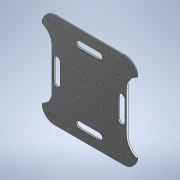
# Autodesk Inventor part: payload_bay_square_FC
Saved by Autodesk Inventor 2022 (Build 260153000, 153)
## iProperties
Created: 2020-02-18
Part Number: payload_bay_square_FC
Material: ABS Plastic
Document SubType Name: Modeling
Designer: Krishna Makhija
Density: 1.06 g/cm^3
Appearance: Smooth - White
Author: Krishna Makhija
Autodesk Inventor part; units mm, degrees
ref_plane "YZ Plane" through (0, 0, 0) normal (1, 0, 0) x (0, 1, 0)
ref_plane "XZ Plane" through (0, 0, 0) normal (0, 1, 0) x (-1, 0, 0)
ref_plane "XY Plane" through (0, 0, 0) normal (0, 0, 1) x (1, 0, 0)
sketch "Sketch1" plane through (0, 0, 0) normal (0, 0, 1) x (1, 0, 0)
  point P0 (0, 0)
sketch "Sketch2" plane through (0, 0, 0) normal (0, 0, 1) x (1, 0, 0)
  line L0 (94.9998, -95.0001) -> (-94.9998, -95.0001)
  line L1 (-94.9998, -95.0001) -> (-94.9998, 95.0001)
  line L2 (-94.9998, 95.0001) -> (94.9998, 95.0001)
  line L3 (94.9998, 95.0001) -> (94.9998, -95.0001)
  line L4 (94.9998, -95.0001) -> (-94.9998, 95.0001) construction
  line L5 (-94.9998, -95.0001) -> (94.9998, 95.0001) construction
  point P0 (0, 0)
  constraints: 12 end point, 2 midpoint, 2 parallel, 1 horizontal, 1 perpendicular
extrude "Extrusion1" add sketch "Sketch2" along normal blind 3
sketch "Sketch3" plane through (0, 0, 3) normal (0, 0, 1) x (1, 0, 0)
  circle A0 centre (70, 80) radius 1.5001
  circle A1 centre (70, -80) radius 1.5001
  circle A2 centre (-70, 80) radius 1.5001
  circle A3 centre (-70, -80) radius 1.5001
  constraints: 4 centre point
extrude "Extrusion2" cut sketch "Sketch3" against normal blind 3
fillet "Fillet1" radius 25 1 edges at (94.9998, 95.0001, 1.5)
fillet "Fillet2" radius 25 1 edges at (94.9998, -95.0001, 1.5)
fillet "Fillet3" radius 25 1 edges at (-94.9998, -95.0001, 1.5)
fillet "Fillet4" radius 25 1 edges at (-94.9998, 95.0001, 1.5)
sketch "Pi mount holes" plane through (0, 0, 3) normal (0, 0, 1) x (1, 0, 0)
  circle A0 centre (24, -30.5) radius 1.2502
  circle A1 centre (-34, -30.5) radius 1.2502
  circle A2 centre (-34, -79.5) radius 1.2502
  circle A3 centre (24, -79.5) radius 1.2502
  constraints: 4 centre point
sketch "B205 mount holes" plane through (0, 0, 3) normal (0, 0, 1) x (1, 0, 0)
  circle A0 centre (20.32, 30.48) radius 1.5002
  circle A1 centre (-45.72, 30.48) radius 1.5002
  circle A2 centre (-45.72, -12.7) radius 1.5002
  circle A3 centre (20.32, -12.7) radius 1.5002
  constraints: 4 centre point
sketch "RM3100 mount holes" plane through (0, 0, 3) normal (0, 0, 1) x (1, 0, 0)
  circle A0 centre (0, 9) radius 0.9999
  circle A1 centre (0, -9) radius 0.9999
  constraints: 2 centre point
sketch "Pololu mount holes" plane through (0, 0, 3) normal (0, 0, 1) x (1, 0, 0)
  circle A0 centre (59.5, 87.75) radius 1.2501
  circle A1 centre (44.5, 87.75) radius 1.2501
  circle A2 centre (44.5, 52.25) radius 1.2501
  circle A3 centre (59.5, 52.25) radius 1.2501
  circle A4 centre (-42.5, -52.25) radius 1.2501
  circle A5 centre (-57.5, -52.25) radius 1.2501
  circle A6 centre (-57.5, -87.75) radius 1.2501
  circle A7 centre (-42.5, -87.75) radius 1.2501
  constraints: 8 centre point
sketch "B205 cable cutout" plane through (0, 0, 3) normal (0, 0, 1) x (1, 0, 0)
  line L0 (-76.0426, -14.5593) -> (-76.0426, 37.4411) construction
  line L1 (-81.5424, -9.0595) -> (-81.5424, 31.9413)
  line L2 (-70.5428, 31.9413) -> (-70.5428, -9.0595)
  arc A0 (-81.5424, -9.0595) -> (-70.5428, -9.0595) centre (-76.0426, -9.0595) ccw
  arc A1 (-70.5428, 31.9413) -> (-81.5424, 31.9413) centre (-76.0426, 31.9413) ccw
  point P0 (0, 0)
  point P1 (-76.0426, 11.4409)
  constraints: 8 end point, 6 point on circle, 4 tangent, 2 centre point, 2 point on line, 1 midpoint, 1 parallel, 1 vertical
sketch "Pi cable cutout" plane through (0, 0, 3) normal (0, 0, 1) x (1, 0, 0)
  line L0 (65.7382, -60.7056) -> (65.7382, 5.2939) construction
  line L1 (60.7378, -55.7052) -> (60.7378, 0.2935)
  line L2 (70.7387, 0.2935) -> (70.7387, -55.7052)
  arc A0 (60.7378, -55.7052) -> (70.7387, -55.7052) centre (65.7382, -55.7052) ccw
  arc A1 (70.7387, 0.2935) -> (60.7378, 0.2935) centre (65.7382, 0.2935) ccw
  point P0 (0, 0)
  point P1 (65.7382, -27.7058)
  constraints: 8 end point, 6 point on circle, 4 tangent, 2 centre point, 2 point on line, 1 midpoint, 1 parallel, 1 vertical
sketch "Imperial standoffs" plane through (0, 0, 3) normal (0, 0, 1) x (1, 0, 0)
  circle A0 centre (80, 80) radius 1.4302
  circle A1 centre (-80, -80) radius 1.4302
  circle A2 centre (80, -80) radius 1.4302
  circle A3 centre (-80, 80) radius 1.4302
  constraints: 4 centre point
extrude "Bottom payload mount holes" cut sketch "Imperial standoffs" against normal blind 10
sketch "FC mount" plane through (0, 0, 3) normal (0, 0, 1) x (1, 0, 0)
  circle A0 centre (-22.5, 22.5) radius 1.4999
  circle A1 centre (-22.5, -22.5) radius 1.4999
  circle A2 centre (22.5, -22.5) radius 1.4999
  circle A3 centre (22.5, 22.5) radius 1.4999
  circle A4 centre (-10.75, 13.75) radius 1.2498
  circle A5 centre (-10.75, -7.75) radius 1.2498
  circle A6 centre (10.75, -7.75) radius 1.2498
  circle A7 centre (10.75, 13.75) radius 1.2498
  point P0 (0, 0)
  constraints: 8 centre point
sketch "FC cable cutouts" plane through (0, 0, 3) normal (0, 0, 1) x (1, 0, 0)
  line L0 (-65, -20.0003) -> (-65, 20.0003) construction
  line L1 (-58.4981, -20.0003) -> (-58.4981, 20.0003)
  line L2 (-71.5019, 20.0003) -> (-71.5019, -20.0003)
  arc A0 (-71.5019, -20.0003) -> (-58.4981, -20.0003) centre (-65, -20.0003) ccw
  arc A1 (-58.4981, 20.0003) -> (-71.5019, 20.0003) centre (-65, 20.0003) ccw
  line L3 (65, -20.0003) -> (65, 20.0003) construction
  line L4 (71.5019, -20.0003) -> (71.5019, 20.0003)
  line L5 (58.4981, 20.0003) -> (58.4981, -20.0003)
  arc A2 (58.4981, -20.0003) -> (71.5019, -20.0003) centre (65, -20.0003) ccw
  arc A3 (71.5019, 20.0003) -> (58.4981, 20.0003) centre (65, 20.0003) ccw
  arc A4 (-20.0003, 76.5019) -> (-20.0003, 63.4981) centre (-20.0003, 70) ccw
  line L6 (-20.0003, 63.4981) -> (20.0003, 63.4981)
  line L7 (20.0003, 70) -> (-20.0003, 70) construction
  line L8 (20.0003, 76.5019) -> (-20.0003, 76.5019)
  arc A5 (20.0003, 63.4981) -> (20.0003, 76.5019) centre (20.0003, 70) ccw
  line L9 (20.0003, -63.4981) -> (-20.0003, -63.4981)
  line L10 (20.0003, -70) -> (-20.0003, -70) construction
  line L11 (-20.0003, -76.5019) -> (20.0003, -76.5019)
  arc A6 (20.0003, -76.5019) -> (20.0003, -63.4981) centre (20.0003, -70) ccw
  arc A7 (-20.0003, -63.4981) -> (-20.0003, -76.5019) centre (-20.0003, -70) ccw
  point P0 (0, 0)
  constraints: 32 end point, 16 point on circle, 16 tangent, 8 centre point, 4 parallel
sketch "Skid cutouts" plane through (0, 0, 3) normal (0, 0, 1) x (1, 0, 0)
  line L0 (75, 0) -> (75, 39.9996)
  line L1 (75, 39.9996) -> (75, 0)
  line L2 (75, 0) -> (75, -40)
  line L3 (94.9998, -70.0001) -> (94.9998, 70.0001) projected
  arc A0 (94.9998, 70.0001) -> (75, 39.9996) centre (106.9986, 40.3344) ccw
  arc A1 (69.9998, -95.0001) -> (94.9998, -70.0001) centre (69.9998, -70.0001) ccw projected
  arc A2 (75, -40) -> (94.9998, -70.0001) centre (106.9987, -40.3344) ccw
  line L4 (-75, 0) -> (-75, -39.9996)
  line L5 (-75, -39.9996) -> (-75, 0)
  line L6 (-75, 0) -> (-75, 40)
  arc A3 (-94.9998, -70.0001) -> (-75, -39.9996) centre (-106.9986, -40.3344) ccw
  arc A4 (-75, 40) -> (-94.9998, 70.0001) centre (-106.9987, 40.3344) ccw
  line L7 (-94.9998, 70.0001) -> (-94.9998, -70.0001) projected
  line L8 (-94.9998, -70.0001) -> (-94.9998, 70.0001)
  line L9 (-94.9998, 70.0001) -> (-94.9998, -70.0001)
  point P0 (0, 0)
  constraints: 16 end point, 8 point on circle, 4 centre point, 4 collinear, 2 vertical
extrude "Extrusion10" cut sketch "Skid cutouts" against normal blind 10
extrude "Extrusion11" cut sketch "FC cable cutouts" against normal blind 10
extrude "Extrusion12" cut sketch "Pololu mount holes" against normal blind 10
extrude "Extrusion13" cut sketch "FC mount" against normal blind 10
body "Solid1"
